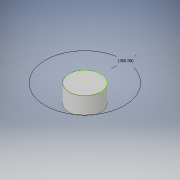
# Autodesk Inventor part: Container Cap test
Saved by Autodesk Inventor 2019 (Build 230136000, 136)
## iProperties
Created: 2019-01-22
Part Number: Container Cap test
Material: Generic
Document SubType Name: Modeling
Designer: pepin
Density: 1 g/cm^3
Appearance: Default
Author: pepin
Autodesk Inventor part; units mm, degrees
ref_plane "YZ Plane" through (0, 0, 0) normal (1, 0, 0) x (0, 1, 0)
ref_plane "XZ Plane" through (0, 0, 0) normal (0, 1, 0) x (-1, 0, 0)
ref_plane "XY Plane" through (0, 0, 0) normal (0, 0, 1) x (1, 0, 0)
sketch "Sketch1" plane through (0, 0, 0) normal (0, 1, 0) x (-1, 0, 0)
  circle A0 centre (0, 0) radius 2.2912
  constraints: 1 centre point, 1 coincident
extrude "Extrusion1" add sketch "Sketch1" along normal blind 2.54
sketch "Sketch2" plane through (0, 2.54, 0) normal (0, 1, 0) x (1, 0, 0)
  line L0 (0.0828, 2.2579) -> (-0.1064, 2.2579)
  line L1 (-0.1064, 2.2579) -> (-0.1064, 2.1752)
  line L2 (-0.1064, 2.1752) -> (0.0828, 2.1752)
  line L3 (0.0828, 2.1752) -> (0.0828, 2.2579)
  line L4 (-0.2715, 2.2431) -> (-0.4583, 2.2135)
  line L5 (-0.619, 2.173) -> (-0.7989, 2.1145)
  line L6 (-0.9513, 2.0494) -> (-1.1199, 1.9635)
  line L7 (-1.2602, 1.8753) -> (-1.4133, 1.7642)
  line L8 (-1.5381, 1.6551) -> (-1.6718, 1.5214)
  line L9 (-1.7781, 1.3941) -> (-1.8892, 1.2411)
  line L10 (-1.9743, 1.0988) -> (-2.0601, 0.9303)
  line L11 (-2.1218, 0.7764) -> (-2.1803, 0.5966)
  line L12 (-2.2172, 0.435) -> (-2.2468, 0.2481)
  line L13 (-2.2579, 0.0828) -> (-2.2579, -0.1064)
  line L14 (-2.2431, -0.2715) -> (-2.2135, -0.4583)
  line L15 (-2.173, -0.619) -> (-2.1145, -0.7989)
  line L16 (-2.0494, -0.9513) -> (-1.9635, -1.1199)
  line L17 (-1.8753, -1.2602) -> (-1.7642, -1.4133)
  line L18 (-1.6551, -1.5381) -> (-1.5214, -1.6718)
  line L19 (-1.3941, -1.7781) -> (-1.2411, -1.8892)
  line L20 (-1.0988, -1.9743) -> (-0.9303, -2.0601)
  line L21 (-0.7764, -2.1218) -> (-0.5966, -2.1803)
  line L22 (-0.435, -2.2172) -> (-0.2481, -2.2468)
  line L23 (-0.0828, -2.2579) -> (0.1064, -2.2579)
  line L24 (0.2715, -2.2431) -> (0.4583, -2.2135)
  line L25 (0.619, -2.173) -> (0.7989, -2.1145)
  line L26 (0.9513, -2.0494) -> (1.1199, -1.9635)
  line L27 (1.2602, -1.8753) -> (1.4133, -1.7642)
  line L28 (1.5381, -1.6551) -> (1.6718, -1.5214)
  line L29 (1.7781, -1.3941) -> (1.8892, -1.2411)
  line L30 (1.9743, -1.0988) -> (2.0601, -0.9303)
  line L31 (2.1218, -0.7764) -> (2.1803, -0.5966)
  line L32 (2.2172, -0.435) -> (2.2468, -0.2481)
  line L33 (2.2579, -0.0828) -> (2.2579, 0.1064)
  line L34 (2.2431, 0.2715) -> (2.2135, 0.4583)
  line L35 (2.173, 0.619) -> (2.1145, 0.7989)
  line L36 (2.0494, 0.9513) -> (1.9635, 1.1199)
  line L37 (1.8753, 1.2602) -> (1.7642, 1.4133)
  line L38 (1.6551, 1.5381) -> (1.5214, 1.6718)
  line L39 (1.3941, 1.7781) -> (1.2411, 1.8892)
  line L40 (1.0988, 1.9743) -> (0.9303, 2.0601)
  line L41 (0.7764, 2.1218) -> (0.5966, 2.1803)
  line L42 (0.435, 2.2172) -> (0.2481, 2.2468)
  point P0 (0, 0)
  dimension "d4" = 360
  constraints: 86 end point, 2 parallel, 1 horizontal, 1 perpendicular, 121 other
body "Solid1"
